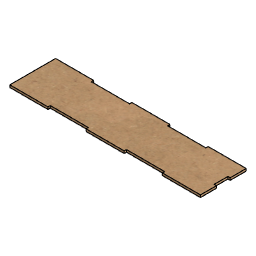
step front v10 (Autodesk Fusion 360 design; units mm, degrees)
Autodesk Fusion 360 part; units mm, degrees
sketch "Sketch1" plane through (0, 0, 0) normal (0, 0, 1) x (1, 0, 0) in component "Step front"
  line L0 (125, 30) -> (-125, 30)
  line L1 (-125, 30) -> (-125, -30)
  line L2 (-125, -30) -> (125, -30)
  line L3 (125, -30) -> (125, 30)
  line L4 (125, 30) -> (-125, -30) construction
  line L5 (-125, 30) -> (125, -30) construction
  line L6 (-125, 30) -> (-75, 30)
  line L7 (-75, 30) -> (-75, 27)
  line L8 (-75, 27) -> (-125, 27)
  line L9 (-125, 27) -> (-125, 30)
  line L10 (-25, 27) -> (-75, 27)
  line L11 (-25, 30) -> (-25, 27)
  line L12 (-75, 30) -> (-25, 30)
  line L13 (-75, 30) -> (-75, -30)
  line L14 (25, 27) -> (-25, 27)
  line L15 (25, 30) -> (25, 27)
  line L16 (-25, 30) -> (25, 30)
  line L17 (-25, 30) -> (-25, -30)
  line L18 (75, 27) -> (25, 27)
  line L19 (75, 30) -> (75, 27)
  line L20 (25, 30) -> (75, 30)
  line L21 (25, 30) -> (25, -30)
  line L22 (125, 27) -> (75, 27)
  line L23 (125, 30) -> (125, 27)
  line L24 (75, 30) -> (125, 30)
  line L25 (75, 30) -> (75, -30)
  line L26 (-75, -30) -> (-125, -30)
  line L27 (-75, -27) -> (-75, -30)
  line L28 (-125, -27) -> (-75, -27)
  line L29 (-125, -27) -> (-125, -30)
  line L30 (-25, -30) -> (-75, -30)
  line L31 (-25, -27) -> (-25, -30)
  line L32 (-75, -27) -> (-25, -27)
  line L33 (-75, -27) -> (-75, -30)
  line L34 (25, -30) -> (-25, -30)
  line L35 (25, -27) -> (25, -30)
  line L36 (-25, -27) -> (25, -27)
  line L37 (-25, -27) -> (-25, -30)
  line L38 (75, -30) -> (25, -30)
  line L39 (75, -27) -> (75, -30)
  line L40 (25, -27) -> (75, -27)
  line L41 (25, -27) -> (25, -30)
  line L42 (125, -30) -> (75, -30)
  line L43 (125, -27) -> (125, -30)
  line L44 (75, -27) -> (125, -27)
  line L45 (75, -27) -> (75, -30)
  dimension "d1" = 250
  dimension "d2" = 60
  dimension "d9" = 50
  dimension "d10" = 3
  constraint horizontal L0
  constraint perpendicular L0 L1
  constraint parallel L0 L2
  constraint parallel L1 L3
  constraint coincident L4 origin
  constraint coincident L5 origin
  constraint horizontal L6
  constraint vertical L7
  constraint horizontal L8
  constraint vertical L9
  measures "d1" distance of L1.end L2.end
  measures "d2" distance of L0.end L1.end
  measures "d9" distance of L0.end L6.end
  measures "d10" distance of L0.end L8.end
extrude "Extrude3" add sketch "Sketch1" along normal blind 3 contours L0 L3 L19 L22 L23 L24 L25 | L3 L22 L25 L44 | L0 L11 L14 L15 L16 L17 L21 | L18 L21 L25 L40 | L2 L3 L25 L39 L42 L43 L44 L45 | L14 L17 L21 L36 | L0 L1 L6 L7 L8 L9 L13 | L10 L13 L17 L32 | L2 L17 L21 L31 L34 L35 L36 L37 L41 | L1 L8 L13 L28 | L1 L2 L13 L26 L27 L28 L29 L33 in component "Step front"
sketch "Sketch3" plane through (0, 0, 3) normal (0, 0, 1) x (-1, 0, 0) in component "Step front"
  line L0 (-25, 27) -> (-75, 27)
  line L1 (-75, 27) -> (-75, 30)
  line L2 (-75, 30) -> (-125, 30)
  line L3 (-125, 30) -> (-125, -30)
  line L4 (-125, -30) -> (-75, -30)
  line L5 (-75, -30) -> (-75, -27)
  line L6 (-75, -27) -> (-25, -27)
  line L7 (-25, -27) -> (-25, -30)
  line L8 (-25, -30) -> (25, -30)
  line L9 (25, -30) -> (25, -27)
  line L10 (25, -27) -> (75, -27)
  line L11 (75, -27) -> (75, -30)
  line L12 (75, -30) -> (125, -30)
  line L13 (125, -30) -> (125, 30)
  line L14 (125, 30) -> (75, 30)
  line L15 (75, 30) -> (75, 27)
  line L16 (75, 27) -> (25, 27)
  line L17 (25, 27) -> (25, 30)
  line L18 (25, 30) -> (-25, 30)
  line L19 (-25, 30) -> (-25, 27)
  line L20 (-125, -30) -> (-122, -30) construction
  line L21 (-122, -30) -> (-122, -8) construction
  line L22 (-122, -8) -> (-125, -8) construction
  line L23 (-125, -8) -> (-125, -30) construction
  line L24 (-125, 30) -> (-122, 30) construction
  line L25 (-122, 30) -> (-122, 8) construction
  line L26 (-122, 8) -> (-125, 8) construction
  line L27 (-125, 8) -> (-125, 30) construction
  line L28 (-125, -9) -> (-122, -9)
  line L29 (-122, -9) -> (-122, 9)
  line L30 (-122, 9) -> (-125, 9)
  line L31 (-125, 9) -> (-125, -9)
  dimension "d17" = 22
  dimension "d18" = 3
  dimension "d19" = 22
  constraint horizontal L20
  constraint vertical L21
  constraint horizontal L22
  constraint vertical L23
  constraint coincident L3.end L4.start
  constraint horizontal L24
  constraint vertical L25
  constraint horizontal L26
  constraint vertical L27
  constraint coincident L2.end L3.start
  constraint horizontal L28
  constraint vertical L29
  constraint horizontal L30
  constraint vertical L31
  constraint coincident L25 L29.end
  constraint coincident L3 L28.start
  measures "d17" distance of L3.end L22.end
  measures "d18" distance of L2.end L24.end
  measures "d19" distance of L2.end L26.end
extrude "Extrude4" cut sketch "Sketch3" against normal blind 12 contours L3 L28 L29 L30 L31 in component "Step front"
sketch "Sketch1 (2)" plane through (0, 0, 3) normal (0, 0, 1) x (-1, 0, 0)
  line L0 (-122, -9) -> (-125, -9)
  line L1 (-125, -9) -> (-125, -30)
  line L2 (-125, -30) -> (-75, -30)
  line L3 (-75, -30) -> (-75, -27)
  line L4 (-75, -27) -> (-25, -27)
  line L5 (-25, -27) -> (-25, -30)
  line L6 (-25, -30) -> (25, -30)
  line L7 (25, -30) -> (25, -27)
  line L8 (25, -27) -> (75, -27)
  line L9 (75, -27) -> (75, -30)
  line L10 (75, -30) -> (125, -30)
  line L11 (125, -30) -> (125, 30)
  line L12 (125, 30) -> (75, 30)
  line L13 (75, 30) -> (75, 27)
  line L14 (75, 27) -> (25, 27)
  line L15 (25, 27) -> (25, 30)
  line L16 (25, 30) -> (-25, 30)
  line L17 (-25, 30) -> (-25, 27)
  line L18 (-25, 27) -> (-75, 27)
  line L19 (-75, 27) -> (-75, 30)
  line L20 (-75, 30) -> (-125, 30)
  line L21 (-125, 30) -> (-125, 9)
  line L22 (-125, 9) -> (-122, 9)
  line L23 (-122, 9) -> (-122, -9)
component "Step front" placed x (1, 0, 0) y (0, 1, 0) z (0, 0, 1) at (0, 0, 0)
